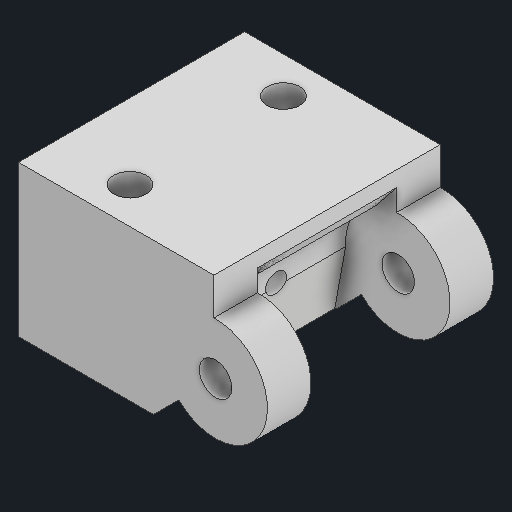
# Autodesk Inventor part: sujeciones_dedos_V13
Saved by Autodesk Inventor 2026.1 (Build 301233020, 233B)
## iProperties
Created: 2026-01-15
Part Number: sujeciones_dedos_V13
Material: Generic
Document SubType Name: Modeling
Designer: user
Density: 1 g/cm^3
Appearance: Default
Author: user
Autodesk Inventor part; units mm, degrees
sketch "Sketch2" plane through (0, 0, 0) normal (0, 0, 1) x (1, 0, 0)
  line L0 (40.7935, -19.9997) -> (-67.2065, -19.9997)
  line L1 (-67.2065, -19.9997) -> (-67.2065, 11.0003)
  circle A0 centre (48.3164, -12.4768) radius 1.575
  arc A1 (44.7809, -16.0123) -> (48.1664, -7.4791) centre (48.3164, -12.4768) ccw
  line L2 (48.1664, 0.0003) -> (48.1664, -7.4791)
  line L3 (48.3164, -12.4768) -> (48.1664, -12.6268)
  line L4 (44.7809, -16.0123) -> (40.7935, -19.9997)
  line L5 (-67.2065, 11.0003) -> (28.1664, 11.0003)
  line L6 (28.1664, 11.0003) -> (48.1664, 0.0003)
  dimension "d19" = 3.15
  dimension "d88" = 10
  dimension "d90" = 0.15
  dimension "d91" = 10.639
  dimension "d111" = 31
  dimension "d135" = 12.4771
  dimension "d176" = 135
  dimension "d177" = 108
  constraints: 14 end point, 2 centre point, 2 perpendicular, 2 point on circle, 1 coincident, 1 parallel, 1 point on line, 1 vertical
  measures "d19" diameter of A0
  measures "d88" diameter of A1
  measures "d90" horizontal distance of A0.centre L2.start
  measures "d91" distance of L0.start A0.centre
  measures "d111" distance of L0.end L1.end
  measures "d135" vertical distance of L2.start A0.centre
  measures "d176" angle of L0 L4
  measures "d177" distance of L0.start L0.end
extrude "Extrusion1" add sketch "Sketch2" along normal mid plane 23
sketch "Sketch5" plane through (0, 0, 0) normal (0, 0, 1) x (1, 0, 0)
  circle A0 centre (48.3164, -12.4768) radius 1.575 projected
  circle A1 centre (48.3164, -12.4768) radius 5.075
  circle A2 centre (48.3164, -12.4768) radius 1.5
  point P0 (0, 0)
  dimension "d28" = 3
  dimension "d29" = 10.15
  constraints: 2 centre point, 2 coincident
  measures "d28" diameter of A2
  measures "d29" diameter of A1
extrude "Extrusion3" cut sketch "Sketch5" along normal mid plane 13.41 contours A1
chamfer "Chamfer2" distance 2 angle 45 1 edges at (48.1664, -7.404, 0)
sketch "Sketch15" plane through (48.1664, -7.4791, -11.5) normal (1, 0, 0) x (0, 0, -1)
  arc A0 (-14.3604, 7.4791) -> (-8.6396, 7.4791) centre (-11.5, 7.4791) ccw
  line L0 (-14.3604, 7.4791) -> (-14.3604, 27.4791)
  line L1 (-14.3604, 27.4791) -> (-8.6396, 27.4791)
  line L2 (-8.6396, 27.4791) -> (-8.6396, 7.4791)
  point P0 (-14.3604, 7.4793)
  point P1 (-11.5, 27.4791)
  dimension "d95" = 5.7208
  dimension "d113" = 20
  constraints: 6 end point, 2 point on circle, 1 centre point, 1 coincident, 1 midpoint, 1 parallel
  measures "d95" diameter of A0
  measures "d113" distance of point (-11.5, 7.479) point (-11.5, 27.479)
sketch "Sketch19" plane through (-67.2065, -19.9997, 11.5) normal (0, -1, 0) x (1, 0, 0)
  line L0 (63.0729, -6) -> (91.3729, -6)
  line L1 (91.3729, -6) -> (91.3729, -19.5)
  line L2 (91.3729, -19.5) -> (63.0729, -19.5)
  line L3 (63.0729, -19.5) -> (63.0729, -6)
  line L4 (63.0729, -6) -> (91.3729, -19.5) construction
  line L5 (91.3729, -6) -> (63.0729, -19.5) construction
  line L6 (115.3729, -18.205) -> (115.3729, -4.795) projected
  line L7 (95.3729, 0) -> (0, 0) projected
  line L8 (108, -23) -> (0, -23) projected
  circle A0 centre (77.2229, -12.75) radius 8.1325
  point P0 (67.2065, -11.5)
  dimension "d104" = 13.5
  dimension "d114" = 24
  dimension "d195" = 28.3
  dimension "d205" = 6
  dimension "d224" = 16.265
  constraints: 12 end point, 2 midpoint, 2 parallel, 1 centre point, 1 coincident, 1 horizontal, 1 perpendicular
  measures "d104" distance of L2.end L0.start
  measures "d114" distance between parallel lines of L6 L1
  measures "d195" distance of L0.start L0.end
  measures "d205" distance between parallel lines of L7 L0
  measures "d224" diameter of A0
extrude "Extrusion13" cut sketch "Sketch19" against normal blind 30 contours L0 A0 L2 L3 | L0 A0 L2 | L0 L1 L2 A0
sketch "Sketch21" plane through (-67.2065, -19.9997, 11.5) normal (0, -1, 0) x (1, 0, 0)
  line L0 (63.0729, -6) -> (91.3729, -6) projected
  line L1 (63.0729, -19.5) -> (63.0729, -6) construction
  line L2 (91.3729, -19.5) -> (63.0729, -19.5) construction
  line L3 (63.0729, -6) -> (91.3729, -19.5)
  line L4 (91.3729, -6) -> (63.0729, -19.5)
  line L5 (95.0229, -19.5) -> (59.4229, -19.5)
  line L6 (59.4229, -19.5) -> (59.4229, -6)
  line L7 (59.4229, -6) -> (95.0229, -6)
  line L8 (95.0229, -6) -> (95.0229, -19.5)
  line L9 (95.0229, -19.5) -> (59.4229, -6) construction
  line L10 (59.4229, -19.5) -> (95.0229, -6) construction
  line L11 (108, -23) -> (108, 0) projected
  point P0 (77.2229, -12.75)
  point P1 (26.7729, -20.5)
  point P2 (26.7729, -7)
  dimension "d164" = 35.6
  dimension "d165" = 13.5
  constraints: 16 end point, 3 midpoint, 2 parallel, 1 horizontal, 1 perpendicular
  measures "d164" distance of L6.end L7.end
  measures "d165" distance of L7.end L5.start
extrude "Extrusion14" cut sketch "Sketch21" against normal blind 10.1
sketch "Sketch20" plane through (-67.2065, 11.0003, 11.5) normal (0, 1, 0) x (1, 0, 0)
  line L0 (115.3729, 23) -> (115.3729, 0) projected
  line L1 (115.3729, 11.5) -> (95.3729, 11.5)
  point P0 (67.2065, 11.5)
  dimension "d107" = 20
  constraints: 2 end point, 1 horizontal, 1 midpoint
  measures "d107" distance of L1.start L1.end
sweep "Sweep3" cut profiles "Sketch15" path "Sketch20" path curves L1
sketch "Sketch22" plane through (48.1664, -7.4791, 11.5) normal (1, 0, 0) x (0, 0, -1)
  circle A0 centre (11.5, -5.0007) radius 1
  line L0 (23, -12.5207) -> (0, -12.5207) projected
  circle A1 centre (11.5, -9.6079) radius 1
  point P0 (11.5, 7.4791)
  dimension "d126" = 7.52
  dimension "d127" = 2.9128
  dimension "d128" = 2
  dimension "d129" = 2
  constraints: 2 centre point
  measures "d126" distance from line of L0 A0.centre
  measures "d127" distance from line of A1.centre L0
  measures "d128" diameter of A1
  measures "d129" diameter of A0
extrude "Extrusion15" cut sketch "Sketch22" against normal through all
ref_plane "Work Plane4" through (48.1664, -2.8604, 0) normal (0, 1, 0) x (-1, 0, 0)
sketch "Sketch26" plane through (48.1664, -2.8604, 0) normal (0, 1, 0) x (-1, 0, 0)
  line L0 (0, -6.705) -> (0, 6.705) projected
  arc A0 (16.24, -0.7321) -> (16.24, 0.7321) centre (16.24, 0) ccw
  line L1 (16.24, -0.7321) -> (0, -0.7321)
  line L2 (16.24, 0.7321) -> (0, 0.7321)
  line L3 (0, 0.7321) -> (0, -0.7321)
  point P0 (48.1664, 0)
  dimension "d147" = 1.4642
  constraints: 6 end point, 2 perpendicular, 2 point on circle, 2 point on line, 1 centre point, 1 collinear, 1 tangent
  measures "d147" diameter of A0
chamfer "Chamfer3" distance 3.6 angle 45 1 edges at (44.7278, -16.0654, 0)
extrude "Extrusion22" add sketch "Sketch26" along normal up to surface surface through (48.1664, 0.0003, 0) normal (0.4819187, 0.8762159, 0)
sketch "Sketch29" plane through (-67.2065, -9.8997, 11.5) normal (0, -1, 0) x (1, 0, 0)
  line L0 (95.0229, -6) -> (95.0229, -19.5) projected
  line L1 (91.3729, -15.7347) -> (95.0229, -15.7347)
  line L2 (95.0229, -15.7347) -> (95.0229, -9.7653)
  line L3 (95.0229, -9.7653) -> (91.3729, -9.7653)
  line L4 (91.3729, -9.7653) -> (91.3729, -15.7347)
  line L5 (91.3729, -19.5) -> (91.3729, -15.7347)
  line L6 (91.3729, -9.7653) -> (91.3729, -6)
  point P0 (67.2065, -11.5)
  dimension "d202" = 3.7653
  dimension "d203" = 3.7653
  constraints: 12 end point, 2 parallel, 1 collinear, 1 horizontal, 1 perpendicular, 1 point on line
  measures "d202" distance of L5.start L1.start
  measures "d203" distance of L3.end L6.end
extrude "Extrusion23" cut sketch "Sketch29" against normal through all
pattern_linear "Rectangular Pattern6" count 2 spacing -31.95 along (1, 0, 0) of "Extrusion23"
pattern_linear "Rectangular Pattern8" count 4 spacing 30 along (0, 0, 1) of "Extrusion1", "Extrusion3", "Chamfer2", "Sweep3", "Extrusion15", "Chamfer3", "Extrusion22"
sketch "Sketch30" plane through (0, 0, 11.5) normal (0, 0, 1) x (1, 0, 0)
  line L0 (48.1664, -7.4791) -> (48.1664, 0.0003) projected
  line L1 (48.1664, 0.0003) -> (28.1664, 11.0003) projected
  line L2 (28.1664, 11.0003) -> (-67.2065, 11.0003) projected
  line L3 (-67.2065, 11.0003) -> (-67.2065, -19.9997) projected
  line L4 (-67.2065, -19.9997) -> (40.7935, -19.9997) projected
  line L5 (40.7935, -19.9997) -> (44.7809, -16.0123) projected
  arc A0 (44.7809, -16.0123) -> (48.1664, -7.4791) centre (48.3164, -12.4768) ccw projected
  circle A1 centre (48.3164, -12.4768) radius 1.575 projected
  circle A2 centre (48.3164, -12.4768) radius 5
  point P0 (0, 0)
  point P1 (28.1664, -19.9997)
  constraints: 1 centre point, 1 coincident, 1 concentric, 1 point on line
extrude "Extrusion24" add sketch "Sketch30" along normal up to surface (7 mm away) contours A2 L5 L4 L3 L2 L1 L0
pattern_linear "Rectangular Pattern9" count 3 spacing 30 along (0, 0, 1) of "Extrusion24"
pattern_linear "Rectangular Pattern10" count 6 spacing 18.5 along (0, 0, 1) of "Extrusion13", "Extrusion14", "Extrusion23", "Rectangular Pattern6"
sketch "Sketch32" plane through (-67.2065, -19.9997, -11.5) normal (0, -1, 0) x (1, 0, 0)
  line L0 (43.9229, 7) -> (57.4229, 7)
  line L1 (57.4229, 7) -> (57.4229, 35.3)
  line L2 (57.4229, 35.3) -> (43.9229, 35.3)
  line L3 (43.9229, 35.3) -> (43.9229, 7)
  line L4 (57.4229, 35.3) -> (43.9229, 7)
  line L5 (57.4229, 7) -> (43.9229, 35.3)
  line L6 (59.4229, 3.5) -> (59.4229, 17) projected
  line L7 (108, 0) -> (0, 0) projected
  point P0 (67.2065, 11.5)
  dimension "d218" = 28.3
  dimension "d219" = 13.5
  dimension "d225" = 2
  dimension "d226" = 7
  constraints: 12 end point, 2 parallel, 1 horizontal, 1 perpendicular
  measures "d218" distance of L2.end L0.start
  measures "d219" distance of L1.end L2.end
  measures "d225" distance between parallel lines of L6 L1
  measures "d226" distance between parallel lines of L0 L7
extrude "Extrusion26" cut sketch "Sketch32" against normal blind 30
sketch "Sketch33" plane through (-67.2065, -19.9997, -11.5) normal (0, -1, 0) x (1, 0, 0)
  line L0 (43.9229, 35.3) -> (57.4229, 35.3) projected
  line L1 (57.4229, 35.3) -> (57.4229, 7) projected
  line L2 (57.4229, 7) -> (43.9229, 7) projected
  line L3 (43.9229, 7) -> (43.9229, 35.3) projected
  line L4 (57.4229, 35.3) -> (43.9229, 7)
  line L5 (57.4229, 7) -> (43.9229, 35.3)
  line L6 (57.4229, 3.35) -> (43.9229, 3.35)
  line L7 (43.9229, 3.35) -> (43.9229, 38.95)
  line L8 (43.9229, 38.95) -> (57.4229, 38.95)
  line L9 (57.4229, 38.95) -> (57.4229, 3.35)
  line L10 (57.4229, 3.35) -> (43.9229, 38.95) construction
  line L11 (43.9229, 3.35) -> (57.4229, 38.95) construction
  point P0 (67.2065, 11.5)
  point P1 (50.6729, 21.15)
  point P2 (57.4229, 7)
  dimension "d240" = 13.5
  dimension "d241" = 35.6
  constraints: 16 end point, 3 midpoint, 2 parallel, 1 horizontal, 1 perpendicular
  measures "d240" distance of L6.start L6.end
  measures "d241" distance of L6.end L7.end
extrude "Extrusion27" cut sketch "Sketch33" against normal blind 10.1
sketch "Sketch34" plane through (-67.2065, -9.8997, -11.5) normal (0, -1, 0) x (1, 0, 0)
  line L0 (57.4229, 3.35) -> (43.9229, 3.35) projected
  line L1 (43.9229, 7) -> (57.4229, 7) projected
  line L2 (57.4229, 7) -> (43.9229, 7) projected
  line L3 (53.6579, 7) -> (47.6879, 7)
  line L4 (47.6879, 7) -> (47.6879, 3.35)
  line L5 (47.6879, 3.35) -> (53.6579, 3.35)
  line L6 (53.6579, 3.35) -> (53.6579, 7)
  line L7 (57.4229, 35.3) -> (57.4229, 7) projected
  line L8 (57.4229, 7) -> (53.6579, 7)
  line L9 (47.6879, 7) -> (43.9229, 7)
  point P0 (67.2065, 11.5)
  point P1 (53.6579, 3.35)
  point P2 (47.6879, 7)
  dimension "d242" = 3.765
  constraints: 12 end point, 3 equal length, 2 horizontal, 2 point on line, 1 collinear, 1 perpendicular
  measures "d242" distance of L1.end L3.start
extrude "Extrusion28" cut sketch "Sketch34" against normal through all
pattern_linear "Rectangular Pattern11" count 2 spacing 31.95 along (0, 0, 1) of "Extrusion28"
pattern_linear "Rectangular Pattern12" count 2 spacing 70.5 along (0, 0, 1) of "Extrusion26", "Extrusion27", "Extrusion28", "Rectangular Pattern11"
ref_plane "Work Plane16" through (-67.2065, -4.4997, 87.6614) normal (0.9396926, 0, 0.3420201) x (0, 1, 0)
sketch "Sketch37" plane through (-67.2065, -4.4997, 87.6614) normal (0.9396926, 0, 0.3420201) x (0, 1, 0)
  line L0 (-15.5, -7.5229) -> (-7.9771, 0) projected
  circle A0 centre (-7.9771, 0.15) radius 4.925
  circle A1 centre (-7.9771, 0.15) radius 1.575
  point P0 (4.4997, -105.3608)
  dimension "d271" = 0.15
  dimension "d272" = 9.85
  dimension "d273" = 3.15
  constraints: 2 centre point, 1 coincident
  measures "d271" distance of A0.centre L0.end
  measures "d272" diameter of A0
  measures "d273" diameter of A1
sketch "Sketch39" plane through (-67.2065, -19.9997, 101.5) normal (0, 0, 1) x (1, 0, 0)
  line L0 (95.3729, 31) -> (0, 31) projected
  line L1 (95.3729, 0) -> (0, 0) projected
  line L2 (0, 31) -> (0, 0) projected
  line L3 (30.3, 0) -> (7, 0)
  line L4 (7, 0) -> (7, 31)
  line L5 (7, 31) -> (30.3, 31)
  line L6 (30.3, 31) -> (30.3, 0)
  point P0 (67.2065, 19.9997)
  point P1 (30.3, 31)
  point P2 (7, 0)
  dimension "d275" = 23.3
  dimension "d276" = 7
  constraints: 8 end point, 2 parallel, 2 point on line, 1 horizontal, 1 perpendicular
  measures "d275" distance of L3.start L3.end
  measures "d276" distance between parallel lines of L2 L4
extrude "Extrusion36" cut sketch "Sketch39" against normal blind 41 contours L6 L1 L4 L0
sketch "Sketch40" plane through (-36.9065, -19.9997, 101.5) normal (-1, 0, 0) x (0, 0, 1)
  line L0 (-41, 31) -> (-41, 0) projected
  line L1 (-41, 15.5) -> (-26, 15.5)
  circle A0 centre (-26, 15.5) radius 15
  circle A1 centre (-26, 15.5) radius 1.575
  point P0 (-101.5, 19.9997)
  dimension "d279" = 15
  dimension "d280" = 30
  dimension "d281" = 3.15
  constraints: 2 centre point, 2 coincident, 2 end point, 1 horizontal, 1 midpoint
  measures "d279" distance of L1.start L1.end
  measures "d280" diameter of A0
  measures "d281" diameter of A1
extrude "Extrusion37" cut sketch "Sketch40" along normal through all contours A1
extrude "Extrusion38" cut sketch "Sketch40" against normal blind 10 contours A1
chamfer "Chamfer5" distance 13.75 angle 45 1 edges at (-36.9065, -4.4997, 101.5)
ref_plane "Work Plane17" through (60.4164, -7.4791, -11.5) normal (1, 0, 0) x (0, 0, -1)
sketch "Sketch41" plane through (60.4164, -7.4791, -11.5) normal (1, 0, 0) x (0, 0, -1)
  line L0 (-0.6, -10.9819) -> (-22.4, -10.9819)
  line L1 (-22.4, -10.9819) -> (-22.4, 3.5681)
  line L2 (-22.4, 3.5681) -> (-0.6, 3.5681)
  line L3 (-0.6, 3.5681) -> (-0.6, -10.9819)
  line L4 (0, -9.9977) -> (0, 0.0023) projected
  line L5 (-18.205, -11.1319) -> (-4.795, -11.1319) projected
  line L6 (-23, 0.0023) -> (-23, -9.9977) projected
  point P0 (-11.5, 7.4791)
  point P1 (0, 0)
  point P2 (0, -8.5333)
  point P3 (-23, -8.5333)
  point P4 (-23, 0)
  dimension "d293" = 14.55
  dimension "d306" = 0.15
  dimension "d307" = 0.6
  dimension "d308" = 0.6
  dimension "d311" = 21.8
  constraints: 8 end point, 2 parallel, 1 horizontal, 1 perpendicular
  measures "d293" distance of L2.end L0.start
  measures "d306" distance between parallel lines of L5 L0
  measures "d307" distance between parallel lines of L4 L3
  measures "d308" distance between parallel lines of L6 L1
  measures "d311" distance of L0.start L0.end
extrude "Extrusion39" cut sketch "Sketch41" against normal blind 31.1 keep common part
sketch "Sketch42" plane through (-67.2065, -19.9997, -11.5) normal (0, -1, 0) x (1, 0, 0)
  circle A0 centre (103.7729, 4.1009) radius 1.575
  line L0 (103.7729, 11.5) -> (97.0263, 11.5)
  circle A1 centre (103.7729, 18.8991) radius 1.575
  point P0 (67.2065, 11.5)
  dimension "d302" = 3.15
  dimension "d303" = 0
  dimension "d309" = 3.15
  dimension "d310" = 7.3991
  constraints: 2 centre point, 2 end point, 1 horizontal, 1 symmetric about line, 1 other
  measures "d302" diameter of A0
  measures "d303" horizontal distance of A0.centre L0.start
  measures "d309" diameter of A1
  measures "d310" distance from line of L0 A0.centre
extrude "Extrusion40" cut sketch "Sketch42" against normal blind 25
ref_plane "Work Plane11" through (48.1664, -2.8604, 30) normal (0, 1, 0) x (-1, 0, 0)
ref_plane "Work Plane12" through (48.1664, -2.8604, 60) normal (0, 1, 0) x (-1, 0, 0)
ref_plane "Work Plane13" through (48.1664, -2.8604, 90) normal (0, 1, 0) x (-1, 0, 0)
equation "\"d88\" = diametroFueraUnion"
equation "\"d90\" = tolerancia"
equation "\"d28\" = diametroDentroUnion"
equation "\"d29\" = diametroFueraUnion + tolerancia"
equation "\"d10\" = 10.639"
equation "\"d16\" = 135deg"
equation "\"d26\" = 135deg"
equation "\"d27\" = 135deg"
equation "\"d30\" = 135deg"
equation "\"d34\" = 23"
equation "\"d35\" = 0"
equation "\"d40\" = 135deg"
equation "\"d41\" = 10.639"
equation "\"d42\" = 11.8875"
equation "\"d43\" = 0"
equation "\"diametroDentroUnion\" = 3"
equation "\"diametroFueraUnion\" = 10"
equation "\"d45\" = 15"
equation "\"d39\" = diametroDentroUnion"
equation "\"anchoServo\" = 12.2"
equation "\"tolerancia\" = 0.15"
equation "\"d193\" = 0.15"
equation "\"d199\" = 0.15"
equation "\"d215\" = 0.15"
equation "\"d216\" = 0.15"
equation "\"servoLargo\" = 28"
equation "\"servoLargoConOrejas\" = 35.3"
equation "\"servoAncho\" = 13.2"
equation "\"ServoAlto\" = 29.7"
equation "\"diametroPolea\" = 16.265"
body "Solid1"
